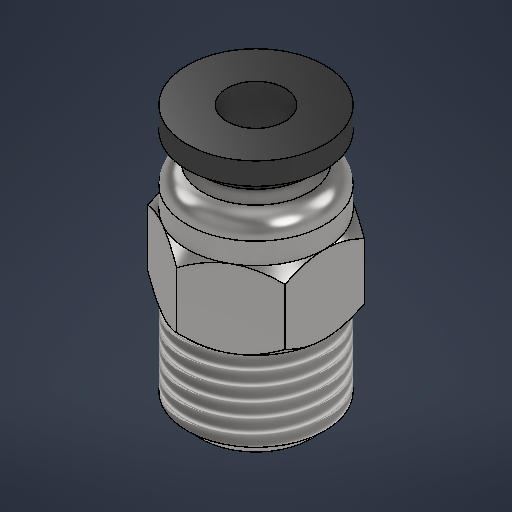
# Autodesk Inventor part: PC4-M10
Saved by Autodesk Inventor 2026.1 (Build 301233020, 233B)
## iProperties
Created: 2025-11-11
Part Number: PC4-M10
Material: Stainless Steel
Document SubType Name: Modeling
Designer: JoshuaEah
Density: 8 g/cm^3
Appearance: Semi-Polished
Author: JoshuaEah
Autodesk Inventor part; units mm, degrees
ref_plane "YZ Plane" through (0, 0, 0) normal (1, 0, 0) x (0, 1, 0)
sketch "PC4 Body Profile" plane through (0, 0, 0) normal (0, 1, 0) x (-1, 0, 0)
  circle A0 centre (5, -2.8868) radius 5
  line L0 (5, -8.6603) -> (0, -5.7735)
  line L1 (0, -5.7735) -> (0, 0)
  line L2 (0, 0) -> (5, 2.8868)
  line L3 (5, 2.8868) -> (10, 0)
  line L4 (10, 0) -> (10, -5.7735)
  line L5 (10, -5.7735) -> (5, -8.6603)
  dimension "d4" = 10
  constraints: 12 end point, 2 coincident, 1 centre point, 1 tangent, 13 other
  measures "d4" diameter of A0
extrude "Extrusion1" add sketch "PC4 Body Profile" along normal blind 5.65
extrude "Extrusion2" add sketch "PC4 Body Profile" against normal blind 6.8 contours A0
extrude "Extrusion3" add sketch "PC4 Body Profile" along normal blind 3 from surface at 5.65 contours A0
sketch "Sketch3" plane through (-5, 8.65, -2.8868) normal (0, 1, 0) x (1, 0, 0)
  circle A0 centre (0, 0) radius 5 projected
  circle A1 centre (0, 0) radius 3.85
  dimension "d28" = 7.7
  constraints: 1 centre point, 1 coincident
  measures "d28" diameter of A1
extrude "Extrusion4" add sketch "Sketch3" along normal blind 1 contours A1
fillet "Fillet1" radius 1.5 1 edges at (0, 8.65, -2.8868)
ref_plane "Work Plane1" through (-2.5, 0, -4.3301) normal (0.5, 0, 0.8660254) x (0.8660254, 0, -0.5)
sketch "Sketch4" plane through (-2.5, 0, -4.3301) normal (0.5, 0, 0.8660254) x (0.8660254, 0, -0.5)
  line L0 (-8.6603, 0) -> (-8.6603, 5.65) projected
  line L1 (2.8868, 0) -> (2.8868, 5.65) projected
  line L2 (-8.6603, 5.65) -> (2.8868, 5.65)
  line L3 (2.8868, 5.65) -> (2.8868, 0)
  line L4 (2.8868, 0) -> (-8.6603, 0)
  line L5 (-8.6603, 0) -> (-8.6603, 5.65)
  line L6 (-2.8868, 5.65) -> (-2.8868, 0)
  line L7 (2.1132, 5.65) -> (2.1132, 0)
  line L8 (2.1132, 5.65) -> (2.8868, 4.8765)
  line L9 (2.1132, 0) -> (2.8868, 0.7735)
  point P0 (2.8868, 4.8765)
  dimension "d32" = 10
  dimension "d33" = 45
  dimension "d34" = 45
  constraints: 16 end point, 4 point on line, 2 midpoint, 2 parallel, 2 perpendicular, 1 horizontal
  measures "d32" diameter of L7 L6
  measures "d33" angle of L2 L8
  measures "d34" angle of L4 L9
revolve "Revolution1" cut sketch "Sketch4" angle 360 about axis through (-5, 5.65, -2.8868) along (0, -1, 0) contours L9 L1 L4 | L2 L1 L8
ref_plane "Work Plane2" through (-5, 10.65, -2.8868) normal (0, 1, 0) x (1, 0, 0)
sketch "PC4 Holes" plane through (-5, -6.8, -2.8868) normal (0, -1, 0) x (1, 0, 0)
  circle A0 centre (0, 0) radius 5 projected
  circle A1 centre (0, 0) radius 3.25
  dimension "d9" = 6.5
  constraints: 1 centre point, 1 coincident
  measures "d9" diameter of A1
sketch "Sketch8" plane through (-5, 9.65, -2.8868) normal (0, 1, 0) x (1, 0, 0)
  circle A0 centre (0, 0) radius 3.85 construction
  circle A1 centre (0, 0) radius 2.9
  dimension "d55" = 5.8
  constraints: 1 centre point, 1 coincident
  measures "d55" diameter of A1
hole "Collet Bore" at (-5, 9.65, -2.8868) direction (0, -1, 0) diameter 5.8 depth 5.4
hole "Rear Bore" at (-5, -6.8, -2.8868) direction (0, 1, 0) diameter 6.5 depth 4
hole "Thru Hole" at (-5, -6.8, -2.8868) direction (0, 1, 0) diameter 4.8 end through all
thread "M10x1" size "M10x1" class "6g" standard "ANSI Metric M Profile" full length
sketch "Collet Profile" plane through (-5, 10.65, -2.8868) normal (0, 1, 0) x (1, 0, 0)
  circle A0 centre (0, 0) radius 3.85 construction
  circle A1 centre (0, 0) radius 2.8
  circle A2 centre (0, 0) radius 5
  dimension "d40" = 5.6
  dimension "d41" = 10
  constraints: 2 centre point, 2 coincident
  measures "d40" diameter of A1
  measures "d41" diameter of A2
extrude "Extrusion5" add sketch "Collet Profile" along normal blind 1.6 separate body contours A1 | A2
extrude "Extrusion6" add sketch "Collet Profile" against normal blind 5.4 contours A1 bodies 2
sketch "Sketch7" plane through (-5, 12.25, -2.8868) normal (0, 1, 0) x (1, 0, 0)
  circle A0 centre (0, 0) radius 5 construction
hole "Collet Thru Hole" at (-5, 12.25, -2.8868) direction (0, -1, 0) diameter 4.2 end through all bodies 2
chamfer "Chamfer1" distance 1 angle 45 1 edges at (0, -6.8, -2.8868)
equation "\"d56\" = d55"
